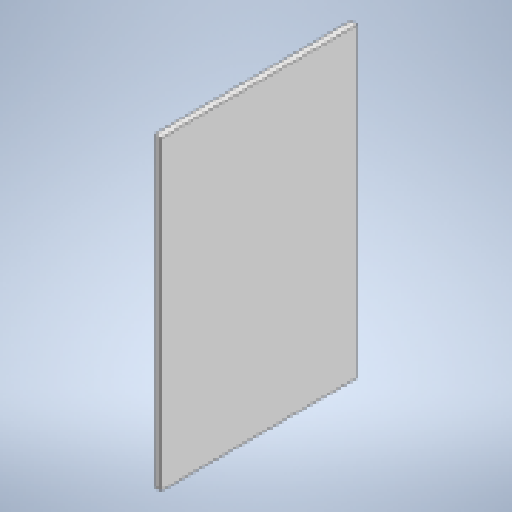
# Autodesk Inventor part: Flat_Plate
Saved by Autodesk Inventor 2023 (Build 270158000, 158)
## iProperties
Created: 2022-05-04
Part Number: Flat_Plate
Material: Generic
Document SubType Name: Modeling
Designer: plebbb
Density: 1 g/cm^3
Appearance: Default
Author: plebbb
Autodesk Inventor part; units mm, degrees
ref_plane "YZ Plane" through (0, 0, 0) normal (1, 0, 0) x (0, 1, 0)
ref_plane "XZ Plane" through (0, 0, 0) normal (0, 1, 0) x (-1, 0, 0)
ref_plane "XY Plane" through (0, 0, 0) normal (0, 0, 1) x (1, 0, 0)
sketch "Sketch1" plane through (0, 0, 0) normal (1, 0, 0) x (0, 1, 0)
  line L0 (0, 0) -> (237.8, 0)
  line L1 (237.8, 0) -> (237.8, -152.4)
  line L2 (237.8, -152.4) -> (0, -152.4)
  line L3 (0, -152.4) -> (0, 0)
  dimension "d0" = 152.4
  dimension "d1" = 237.8
  constraints: 8 end point, 2 parallel, 1 coincident, 1 horizontal, 1 perpendicular
  measures "d0" distance of L0.end L1.end
  measures "d1" distance of L1.end L2.end
extrude "Extrusion1" add sketch "Sketch1" along normal blind 5.08
sketch "Sketch2" plane through (5.08, 0, 0) normal (1, 0, 0) x (0, 0, -1)
  line L0 (53.2, 10) -> (99.2, 10) construction
  line L1 (99.2, 10) -> (99.2, 35) construction
  line L2 (99.2, 35) -> (53.2, 35) construction
  line L3 (53.2, 35) -> (53.2, 10) construction
  circle A0 centre (53.2, 10) radius 4
  circle A1 centre (99.2, 10) radius 4
  circle A2 centre (53.2, 35) radius 4
  circle A3 centre (99.2, 35) radius 4
  line L4 (0, 0) -> (152.4, 0) construction
  point P0 (76.2, 10)
  point P1 (76.2, 0)
  dimension "d4" = 8
  dimension "d5" = 46
  dimension "d6" = 25
  dimension "d7" = 10
  constraints: 8 end point, 4 centre point, 4 coincident, 3 equal radius, 2 midpoint, 2 parallel, 1 horizontal, 1 perpendicular, 1 vertical alignment
  measures "d4" diameter of A0
  measures "d5" distance of L0.start L0.end
  measures "d6" distance of L2.end L0.start
  measures "d7" distance between parallel lines of L4 L0
extrude "Extrusion2" cut sketch "Sketch2" against normal blind 5.08
body "Solid1"
